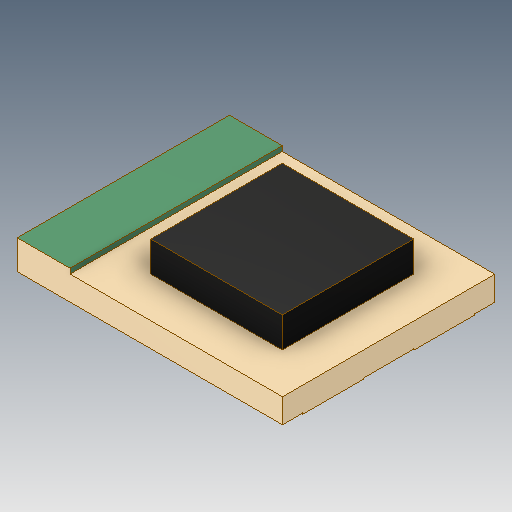
# Autodesk Inventor part: mppc
Saved by Autodesk Inventor 2018.2 (Build 222227000, 227)
## iProperties
Created: 2016-03-28
Part Number: mppc
Material: ABS Plastic
Document SubType Name: Modeling
Designer: sawai
Density: 1.06 g/cm^3
Appearance: Smooth - Off-White
Author: sawai
Autodesk Inventor part; units mm, degrees
ref_plane "YZ Plane" through (0, 0, 0) normal (1, 0, 0) x (0, 1, 0)
ref_plane "XZ Plane" through (0, 0, 0) normal (0, 1, 0) x (-1, 0, 0)
ref_plane "XY Plane" through (0, 0, 0) normal (0, 0, 1) x (1, 0, 0)
sketch "Sketch1" plane through (0, 0, 0) normal (0, 1, 0) x (-1, 0, 0)
  line L0 (1.3125, 1.05) -> (-1.3125, 1.05)
  line L1 (-1.3125, 1.05) -> (-1.3125, -1.05)
  line L2 (-1.3125, -1.05) -> (1.3125, -1.05)
  line L3 (1.3125, -1.05) -> (1.3125, 1.05)
  line L4 (1.3125, 1.05) -> (-1.3125, -1.05) construction
  line L5 (-1.3125, 1.05) -> (1.3125, -1.05) construction
  point P0 (0, 0)
  dimension "d0" = 2.625
  dimension "d1" = 2.1
  constraints: 12 end point, 2 midpoint, 2 parallel, 1 horizontal, 1 perpendicular
  measures "d0" distance of L2.end L1.end
  measures "d1" distance of L1.end L0.end
extrude "Extrusion1" add sketch "Sketch1" along normal blind 0.85
sketch "Sketch2" plane through (0, 0.85, 0) normal (0, 1, 0) x (1, 0, 0)
  line L0 (-0.39, -0.65) -> (0.91, -0.65)
  line L1 (0.91, -0.65) -> (0.91, 0.65)
  line L2 (0.91, 0.65) -> (-0.39, 0.65)
  line L3 (-0.39, 0.65) -> (-0.39, -0.65)
  line L4 (-0.39, -0.65) -> (0.91, 0.65) construction
  line L5 (0.91, -0.65) -> (-0.39, 0.65) construction
  line L6 (-1.3125, -1.05) -> (1.3125, -1.05) projected
  line L7 (1.3125, -1.05) -> (1.3125, 1.05) projected
  line L8 (1.3125, 1.05) -> (-1.3125, 1.05) projected
  line L9 (-1.3125, 1.05) -> (-1.3125, -1.05) projected
  point P0 (0, 0)
  point P1 (0.26, 0)
  dimension "d4" = 0.26
  dimension "d5" = 1.3
  dimension "d6" = 1.3
  dimension "d7" = 0
  constraints: 12 end point, 2 midpoint, 2 parallel, 1 horizontal, 1 perpendicular
  measures "d4" distance of point (0, 0) point (0.26, 0)
  measures "d5" distance of L0.end L1.end
  measures "d6" distance of L1.end L2.end
  measures "d7" vertical distance of point (0, 0) point (0.26, 0)
extrude "Extrusion2" cut sketch "Sketch2" against normal blind 0.3 contours L3 L2 L1 L0
sketch "Sketch3" plane through (0, 0.85, 0) normal (0, 1, 0) x (1, 0, 0)
  line L0 (0.91, 0.65) -> (0.91, -0.65) projected
  line L1 (0.91, -0.65) -> (-0.39, -0.65) projected
  line L2 (-0.39, -0.65) -> (-0.39, 0.65) projected
  line L3 (-0.39, 0.65) -> (0.91, 0.65) projected
  line L4 (-1.3125, -1.05) -> (1.3125, -1.05) projected
  line L5 (1.3125, -1.05) -> (1.3125, 1.05) projected
  line L6 (1.3125, 1.05) -> (-1.3125, 1.05) projected
  line L7 (-1.3125, 1.05) -> (-1.3125, -1.05) projected
  point P0 (0, 0)
extrude "Extrusion3" cut sketch "Sketch3" against normal blind 0.6
sketch "Sketch4" plane through (0, 0.25, 0) normal (0, 1, 0) x (1, 0, 0)
  line L0 (0.91, 0.65) -> (-0.39, 0.65) projected
  line L1 (0.91, -0.65) -> (0.91, 0.65) projected
  line L2 (-0.39, -0.65) -> (0.91, -0.65) projected
  line L3 (-0.39, 0.65) -> (-0.39, -0.65) projected
  line L4 (1.3125, -1.05) -> (-1.3125, -1.05) projected
  line L5 (1.3125, 1.05) -> (1.3125, -1.05) projected
  line L6 (-1.3125, 1.05) -> (1.3125, 1.05) projected
  line L7 (-1.3125, -1.05) -> (-1.3125, 1.05) projected
  line L8 (1.3125, 1.05) -> (-1.3125, 1.05) projected
  line L9 (-0.79, 1.05) -> (-0.79, -1.05)
  line L10 (1.3125, -1.05) -> (-1.3125, -1.05) projected
  point P0 (0, 0)
  dimension "d12" = 0.4
  constraints: 2 end point, 2 point on line, 1 perpendicular
  measures "d12" distance between parallel lines of L3 L9
extrude "Extrusion4" add sketch "Sketch4" along normal blind 0.05 contours L4 L7 L6 L9
sketch "Sketch5" plane through (0, 0, 0) normal (0, -1, 0) x (1, 0, 0)
  line L0 (-1.3125, 1.05) -> (1.3125, 1.05) projected
  line L1 (-1.3125, -1.05) -> (-1.3125, 1.05) projected
  line L2 (1.3125, -1.05) -> (-1.3125, -1.05) projected
  line L3 (1.3125, 1.05) -> (1.3125, -1.05) projected
  line L4 (1.3125, -1.05) -> (1.3125, 1.05) projected
  line L5 (1.3125, 0.85) -> (0.7125, 0.85)
  line L6 (0.7125, 0.85) -> (0.7125, 0.25)
  line L7 (0.7125, 0.25) -> (1.3125, 0.25)
  line L8 (1.3125, 0.25) -> (1.3125, 0.85)
  line L9 (1.3125, 0) -> (-1.3125, 0) construction
  line L10 (1.3125, 1.05) -> (-0.79, 1.05) projected
  line L11 (0, 1.05) -> (0, -1.05) construction
  line L12 (1.3125, -0.85) -> (0.7125, -0.85)
  line L13 (0.7125, -0.85) -> (0.7125, -0.25)
  line L14 (0.7125, -0.25) -> (1.3125, -0.25)
  line L15 (1.3125, -0.25) -> (1.3125, -0.85)
  line L16 (-1.3125, 1.05) -> (-1.3125, -1.05)
  line L17 (-1.3125, -1.05) -> (-1.3125, 1.05)
  line L18 (-1.3125, 0.85) -> (-0.7125, 0.85)
  line L19 (-0.7125, 0.85) -> (-0.7125, 0.25)
  line L20 (-0.7125, 0.25) -> (-1.3125, 0.25)
  line L21 (-1.3125, 0.25) -> (-1.3125, 0.85)
  line L22 (-1.3125, -0.85) -> (-0.7125, -0.85)
  line L23 (-0.7125, -0.85) -> (-0.7125, -0.25)
  line L24 (-0.7125, -0.25) -> (-1.3125, -0.25)
  line L25 (-1.3125, -0.25) -> (-1.3125, -0.85)
  point P0 (0, 0)
  dimension "d15" = 0.25
  dimension "d16" = 0.6
  dimension "d17" = 0.6
  constraints: 40 end point, 12 symmetric about line, 4 midpoint, 3 point on line, 2 parallel, 1 horizontal, 1 perpendicular
  measures "d15" distance from line of L7 point (0, 0)
  measures "d16" distance of L5.end L6.end
  measures "d17" distance between parallel lines of L3 L6
extrude "Extrusion5" cut sketch "Sketch5" against normal blind 0.01 contours L0 L3 L5 L6 L7 L14 L13 L12 L2 L1 L22 L23 L24 L20 L19 L18
sketch "Sketch6" plane through (0, 0.01, 0) normal (0, -1, 0) x (1, 0, 0)
  circle A0 centre (0, -0.6515) radius 0.05
  point P0 (0, 0)
  dimension "d20" = 0.1
  constraints: 1 centre point
  measures "d20" diameter of A0
extrude "Extrusion6" add sketch "Sketch6" along normal up to surface (0.01 mm away)
body "Solid1"
